Autodesk Fusion 360 part; units mm, degrees
(part 2 of 2)
sketch "スケッチ6" plane through (0, 0, -2.5) normal (0, 0, -1) x (-1, 0, 0)
  line L0 (11.25, 45.9909) -> (-11.25, 45.9909)
  line L1 (-11.25, 45.9909) -> (-11.25, 59.4909)
  line L2 (-11.25, 59.4909) -> (11.25, 59.4909)
  line L3 (11.25, 59.4909) -> (11.25, 45.9909)
  circle A0 centre (7.9, 62.4909) radius 1.5
  circle A1 centre (-7.9, 62.4909) radius 1.5
  line L4 (17.25, 45.9909) -> (17.25, 65.4909)
  line L5 (17.25, 65.4909) -> (-17.25, 65.4909)
  line L6 (-17.25, 65.4909) -> (-17.25, 45.9909)
  line L7 (-17.25, 45.9909) -> (-31.8909, 45.9909)
  line L8 (-31.8909, 45.9909) -> (-31.8909, 81.9198)
  line L9 (-31.8909, 81.9198) -> (-24.8198, 88.9909)
  line L10 (-24.8198, 88.9909) -> (24.8198, 88.9909)
  line L11 (24.8198, 88.9909) -> (31.8909, 81.9198)
  line L12 (31.8909, 81.9198) -> (31.8909, 45.9909)
  line L13 (31.8909, 45.9909) -> (17.25, 45.9909)
  line L14 (24.5921, 31.6632) -> (3.3789, 10.45)
  line L15 (3.3789, 10.45) -> (-3.3789, 10.45)
  line L16 (-3.3789, 10.45) -> (-24.5921, 31.6632)
  line L17 (-24.5921, 31.6632) -> (-24.5921, 38.8909)
  line L18 (-24.5921, 38.8909) -> (24.5921, 38.8909)
  line L19 (24.5921, 38.8909) -> (24.5921, 31.6632)
  line L20 (0, 0) -> (38.8909, 38.8909)
  line L21 (38.8909, 38.8909) -> (38.8909, 95.9909)
  line L22 (38.8909, 95.9909) -> (-38.8909, 95.9909)
  line L23 (-38.8909, 95.9909) -> (-38.8909, 38.8909)
  line L24 (-38.8909, 38.8909) -> (0, 0)
  circle A2 centre (31.8909, 38.8909) radius 3.25
  circle A3 centre (-33.6231, 90.7231) radius 3.25
  circle A4 centre (33.6231, 90.7231) radius 3.25
  circle A5 centre (-31.8909, 38.8909) radius 3.25
  line L25 (10.25, 64.4909) -> (-10.25, 64.4909)
  line L26 (-10.25, 64.4909) -> (-10.25, 49.0909)
  line L27 (-10.25, 49.0909) -> (10.25, 49.0909)
  line L28 (10.25, 49.0909) -> (10.25, 64.4909)
  line L29 (10.25, 64.4909) -> (-10.25, 49.0909) construction
  line L30 (-10.25, 64.4909) -> (10.25, 49.0909) construction
  line L31 (0, 56.7909) -> (0, 0) construction
  point P0 (0, 56.7909)
  dimension "d56" = 20.5
  dimension "d57" = 15.4
  dimension "d58" = 2
  constraint horizontal L25
  constraint perpendicular L25 L26
  constraint parallel L25 L27
  constraint parallel L26 L28
  constraint coincident L29 P0
  constraint coincident L30 P0
  constraint coincident P0 L31.start
  constraint coincident L20.start L24.end
  constraint perpendicular L15 L31
  measures "d56" distance of L25.start L25.end
  measures "d57" distance of L25.start L27.end
  measures "d58" distance of A0.centre L25
extrude "押し出し8" add sketch "スケッチ6" along normal blind 0.79 separate body contours L2 L26 L27 L28 | L2 L25 L26 L28 makes body 2
named bodies: "MPU6050"
